Autodesk Fusion 360 part; units mm, degrees
(part 5 of 6)
  spline S189 degree 5 poles (-34.4509, 30.6181) (-34.451, 30.6199) (-34.4519, 30.6304) (-34.4535, 30.6496) (-34.4558, 30.6774) (-34.4591, 30.7139) (-34.4633, 30.7573) (-34.4677, 30.8007) (-34.4723, 30.8442) (-34.4771, 30.8876) (-34.4821, 30.9311) (-34.4873, 30.9746) (-34.4928, 31.0181) (-34.4985, 31.0616) (-34.5043, 31.1051) (-34.5104, 31.1486) (-34.5167, 31.1922) (-34.5231, 31.2358) (-34.5298, 31.2793) (-34.5367, 31.3229) (-34.5437, 31.3665) (-34.551, 31.4102) (-34.5584, 31.4538) (-34.566, 31.4974) (-34.5738, 31.541) (-34.5818, 31.5847) (-34.59, 31.6283) (-34.5984, 31.672) (-34.6069, 31.7157) (-34.6156, 31.7594) (-34.6245, 31.803) (-34.6336, 31.8467) (-34.6428, 31.8904) (-34.6522, 31.9341) (-34.6618, 31.9778) (-34.6715, 32.0215) (-34.6815, 32.0652) (-34.6916, 32.1089) (-34.7018, 32.1527) (-34.7122, 32.1964) (-34.7228, 32.2401) (-34.7336, 32.2838) (-34.7445, 32.3275) (-34.7556, 32.3713) (-34.7668, 32.415) (-34.7782, 32.4587) (-34.7897, 32.5024) (-34.7991, 32.5374) (-34.8062, 32.5636) (-34.811, 32.5811) (-34.8134, 32.5899) knots 0.354152 0.354152 0.354152 0.354152 0.354152 0.354152 0.357143 0.371429 0.385714 0.4 0.414286 0.428571 0.442857 0.457143 0.471429 0.485714 0.5 0.514286 0.528571 0.542857 0.557143 0.571429 0.585714 0.6 0.614286 0.628571 0.642857 0.657143 0.671429 0.685714 0.7 0.714286 0.728571 0.742857 0.757143 0.771429 0.785714 0.8 0.814286 0.828571 0.842857 0.857143 0.871429 0.885714 0.9 0.914286 0.928571 0.942857 0.957143 0.971429 0.985714 1 1 1 1 1 1
  arc A95 (-34.8134, 32.5899) -> (-35.5172, 32.6941) centre (-40, 0) ccw
  spline S190 degree 5 poles (-35.5172, 32.6941) (-35.5221, 32.6864) (-35.5317, 32.6711) (-35.5461, 32.648) (-35.5652, 32.6173) (-35.5889, 32.5788) (-35.6125, 32.5402) (-35.6359, 32.5016) (-35.6592, 32.463) (-35.6823, 32.4243) (-35.7053, 32.3856) (-35.7281, 32.3468) (-35.7507, 32.308) (-35.7732, 32.2692) (-35.7955, 32.2302) (-35.8177, 32.1913) (-35.8397, 32.1523) (-35.8615, 32.1132) (-35.8832, 32.0741) (-35.9047, 32.035) (-35.9261, 31.9958) (-35.9472, 31.9566) (-35.9682, 31.9173) (-35.9891, 31.878) (-36.0097, 31.8386) (-36.0302, 31.7992) (-36.0505, 31.7598) (-36.0706, 31.7203) (-36.0906, 31.6807) (-36.1103, 31.6411) (-36.1299, 31.6015) (-36.1493, 31.5618) (-36.1685, 31.5221) (-36.1875, 31.4823) (-36.2063, 31.4425) (-36.225, 31.4026) (-36.2434, 31.3627) (-36.2616, 31.3227) (-36.2797, 31.2827) (-36.2975, 31.2427) (-36.3151, 31.2026) (-36.3325, 31.1624) (-36.3497, 31.1222) (-36.3667, 31.082) (-36.3835, 31.0417) (-36.4, 31.0014) (-36.4138, 30.9674) (-36.4241, 30.9414) (-36.4312, 30.9236) (-36.435, 30.9138) (-36.4357, 30.9121) knots -1 -1 -1 -1 -1 -1 -0.985714 -0.971429 -0.957143 -0.942857 -0.928571 -0.914286 -0.9 -0.885714 -0.871429 -0.857143 -0.842857 -0.828571 -0.814286 -0.8 -0.785714 -0.771429 -0.757143 -0.742857 -0.728571 -0.714286 -0.7 -0.685714 -0.671429 -0.657143 -0.642857 -0.628571 -0.614286 -0.6 -0.585714 -0.571429 -0.557143 -0.542857 -0.528571 -0.514286 -0.5 -0.485714 -0.471429 -0.457143 -0.442857 -0.428571 -0.414286 -0.4 -0.385714 -0.371429 -0.357143 -0.354152 -0.354152 -0.354152 -0.354152 -0.354152 -0.354152
  spline S191 degree 3 poles (-36.9506, 30.5976) (-36.8858, 30.5912) (-36.8204, 30.5974) (-36.6956, 30.6347) (-36.6374, 30.6653) (-36.5533, 30.7333) (-36.5234, 30.7646) (-36.4724, 30.8341) (-36.4515, 30.872) (-36.4357, 30.9121) knots 0 0 0 0 0.019532 0.019532 0.039064 0.039064 0.051994 0.051994 0.064924 0.064924 0.064924 0.064924
  arc A96 (-36.9506, 30.5976) -> (-37.0349, 30.6059) centre (-40, 0) ccw
  spline S192 degree 3 poles (-37.4787, 31.0146) (-37.4671, 30.9505) (-37.4431, 30.8893) (-37.373, 30.7796) (-37.3276, 30.7321) (-37.2391, 30.6698) (-37.2008, 30.6497) (-37.12, 30.6197) (-37.0778, 30.6101) (-37.0349, 30.6059) knots 0 0 0 0 0.019532 0.019532 0.039064 0.039064 0.051994 0.051994 0.064924 0.064924 0.064924 0.064924
  spline S193 degree 5 poles (-37.4787, 31.0146) (-37.479, 31.0164) (-37.4809, 31.0267) (-37.4843, 31.0456) (-37.4895, 31.0731) (-37.4963, 31.1091) (-37.5047, 31.1519) (-37.5133, 31.1947) (-37.5221, 31.2374) (-37.5312, 31.2802) (-37.5404, 31.323) (-37.5499, 31.3657) (-37.5596, 31.4085) (-37.5695, 31.4512) (-37.5796, 31.494) (-37.5899, 31.5367) (-37.6004, 31.5795) (-37.6111, 31.6222) (-37.6221, 31.6649) (-37.6332, 31.7076) (-37.6445, 31.7503) (-37.6559, 31.793) (-37.6676, 31.8357) (-37.6795, 31.8784) (-37.6915, 31.921) (-37.7038, 31.9637) (-37.7162, 32.0063) (-37.7288, 32.049) (-37.7415, 32.0916) (-37.7545, 32.1342) (-37.7676, 32.1768) (-37.7809, 32.2194) (-37.7944, 32.262) (-37.808, 32.3045) (-37.8219, 32.3471) (-37.8359, 32.3896) (-37.85, 32.4321) (-37.8643, 32.4746) (-37.8788, 32.5171) (-37.8935, 32.5596) (-37.9083, 32.6021) (-37.9233, 32.6446) (-37.9384, 32.687) (-37.9537, 32.7294) (-37.9692, 32.7718) (-37.9848, 32.8142) (-38.0006, 32.8566) (-38.0134, 32.8905) (-38.023, 32.9159) (-38.0295, 32.9328) (-38.0327, 32.9413) knots 0.354152 0.354152 0.354152 0.354152 0.354152 0.354152 0.357143 0.371429 0.385714 0.4 0.414286 0.428571 0.442857 0.457143 0.471429 0.485714 0.5 0.514286 0.528571 0.542857 0.557143 0.571429 0.585714 0.6 0.614286 0.628571 0.642857 0.657143 0.671429 0.685714 0.7 0.714286 0.728571 0.742857 0.757143 0.771429 0.785714 0.8 0.814286 0.828571 0.842857 0.857143 0.871429 0.885714 0.9 0.914286 0.928571 0.942857 0.957143 0.971429 0.985714 1 1 1 1 1 1
  arc A97 (-38.0327, 32.9413) -> (-38.7434, 32.9761) centre (-40, 0) ccw
  spline S194 degree 5 poles (-38.7434, 32.9761) (-38.7475, 32.968) (-38.7555, 32.9517) (-38.7676, 32.9274) (-38.7836, 32.8949) (-38.8034, 32.8543) (-38.8231, 32.8136) (-38.8427, 32.7729) (-38.862, 32.7322) (-38.8812, 32.6914) (-38.9003, 32.6506) (-38.9192, 32.6098) (-38.9379, 32.5689) (-38.9565, 32.5281) (-38.9749, 32.4872) (-38.9931, 32.4462) (-39.0112, 32.4052) (-39.0291, 32.3642) (-39.0469, 32.3232) (-39.0644, 32.2822) (-39.0818, 32.2411) (-39.099, 32.2) (-39.1161, 32.1588) (-39.133, 32.1176) (-39.1497, 32.0764) (-39.1662, 32.0352) (-39.1825, 31.9939) (-39.1987, 31.9527) (-39.2146, 31.9113) (-39.2304, 31.87) (-39.246, 31.8286) (-39.2614, 31.7872) (-39.2766, 31.7458) (-39.2917, 31.7044) (-39.3065, 31.6629) (-39.3211, 31.6214) (-39.3356, 31.5799) (-39.3498, 31.5383) (-39.3638, 31.4967) (-39.3776, 31.4551) (-39.3912, 31.4135) (-39.4046, 31.3718) (-39.4178, 31.3302) (-39.4308, 31.2885) (-39.4435, 31.2467) (-39.456, 31.205) (-39.4664, 31.1698) (-39.4741, 31.143) (-39.4794, 31.1245) (-39.4823, 31.1144) (-39.4828, 31.1126) knots -1 -1 -1 -1 -1 -1 -0.985714 -0.971429 -0.957143 -0.942857 -0.928571 -0.914286 -0.9 -0.885714 -0.871429 -0.857143 -0.842857 -0.828571 -0.814286 -0.8 -0.785714 -0.771429 -0.757143 -0.742857 -0.728571 -0.714286 -0.7 -0.685714 -0.671429 -0.657143 -0.642857 -0.628571 -0.614286 -0.6 -0.585714 -0.571429 -0.557143 -0.542857 -0.528571 -0.514286 -0.5 -0.485714 -0.471429 -0.457143 -0.442857 -0.428571 -0.414286 -0.4 -0.385714 -0.371429 -0.357143 -0.354152 -0.354152 -0.354152 -0.354152 -0.354152 -0.354152
  spline S195 degree 3 poles (-39.9643, 30.7492) (-39.8992, 30.7491) (-39.8347, 30.7617) (-39.7142, 30.811) (-39.6593, 30.8472) (-39.5822, 30.9231) (-39.5556, 30.9572) (-39.5116, 31.0314) (-39.4946, 31.0712) (-39.4828, 31.1126) knots 0 0 0 0 0.019532 0.019532 0.039064 0.039064 0.051994 0.051994 0.064924 0.064924 0.064924 0.064924
  arc A98 (-39.9643, 30.7492) -> (-40.0491, 30.7492) centre (-40, 0) ccw
  spline S196 degree 3 poles (-40.5308, 31.1124) (-40.513, 31.0498) (-40.4831, 30.9912) (-40.4026, 30.8889) (-40.3527, 30.846) (-40.2586, 30.7928) (-40.2185, 30.7765) (-40.1351, 30.7546) (-40.0922, 30.7491) (-40.0491, 30.7492) knots 0 0 0 0 0.019532 0.019532 0.039064 0.039064 0.051994 0.051994 0.064924 0.064924 0.064924 0.064924
  spline S197 degree 5 poles (-40.5308, 31.1124) (-40.5313, 31.1141) (-40.5342, 31.1242) (-40.5395, 31.1427) (-40.5472, 31.1696) (-40.5576, 31.2047) (-40.5701, 31.2465) (-40.5829, 31.2882) (-40.5959, 31.3299) (-40.6091, 31.3716) (-40.6225, 31.4132) (-40.6361, 31.4549) (-40.6499, 31.4965) (-40.664, 31.538) (-40.6782, 31.5796) (-40.6927, 31.6211) (-40.7073, 31.6626) (-40.7222, 31.7041) (-40.7372, 31.7455) (-40.7524, 31.7869) (-40.7679, 31.8283) (-40.7835, 31.8697) (-40.7993, 31.911) (-40.8153, 31.9523) (-40.8314, 31.9936) (-40.8478, 32.0348) (-40.8643, 32.0761) (-40.8811, 32.1173) (-40.8979, 32.1584) (-40.915, 32.1996) (-40.9322, 32.2407) (-40.9497, 32.2817) (-40.9672, 32.3228) (-40.985, 32.3638) (-41.0029, 32.4048) (-41.021, 32.4458) (-41.0393, 32.4867) (-41.0577, 32.5276) (-41.0763, 32.5685) (-41.095, 32.6093) (-41.1139, 32.6501) (-41.133, 32.6909) (-41.1522, 32.7317) (-41.1716, 32.7724) (-41.1912, 32.8131) (-41.2109, 32.8537) (-41.2308, 32.8944) (-41.2468, 32.9268) (-41.2588, 32.9512) (-41.2669, 32.9674) (-41.271, 32.9755) knots 0.354152 0.354152 0.354152 0.354152 0.354152 0.354152 0.357143 0.371429 0.385714 0.4 0.414286 0.428571 0.442857 0.457143 0.471429 0.485714 0.5 0.514286 0.528571 0.542857 0.557143 0.571429 0.585714 0.6 0.614286 0.628571 0.642857 0.657143 0.671429 0.685714 0.7 0.714286 0.728571 0.742857 0.757143 0.771429 0.785714 0.8 0.814286 0.828571 0.842857 0.857143 0.871429 0.885714 0.9 0.914286 0.928571 0.942857 0.957143 0.971429 0.985714 1 1 1 1 1 1
  arc A99 (-41.271, 32.9755) -> (-41.9817, 32.9404) centre (-40, 0) ccw
  spline S198 degree 5 poles (-41.9817, 32.9404) (-41.9849, 32.932) (-41.9914, 32.915) (-42.001, 32.8896) (-42.0137, 32.8557) (-42.0295, 32.8133) (-42.0451, 32.7709) (-42.0605, 32.7285) (-42.0758, 32.6861) (-42.091, 32.6436) (-42.1059, 32.6012) (-42.1207, 32.5587) (-42.1354, 32.5162) (-42.1498, 32.4737) (-42.1641, 32.4312) (-42.1783, 32.3887) (-42.1922, 32.3461) (-42.206, 32.3036) (-42.2197, 32.261) (-42.2331, 32.2184) (-42.2464, 32.1758) (-42.2595, 32.1332) (-42.2725, 32.0906) (-42.2852, 32.048) (-42.2978, 32.0053) (-42.3102, 31.9627) (-42.3224, 31.92) (-42.3344, 31.8773) (-42.3463, 31.8347) (-42.3579, 31.792) (-42.3694, 31.7493) (-42.3807, 31.7066) (-42.3918, 31.6639) (-42.4027, 31.6211) (-42.4133, 31.5784) (-42.4238, 31.5357) (-42.4341, 31.4929) (-42.4442, 31.4502) (-42.4541, 31.4074) (-42.4638, 31.3647) (-42.4732, 31.3219) (-42.4825, 31.2791) (-42.4915, 31.2364) (-42.5003, 31.1936) (-42.5089, 31.1508) (-42.5173, 31.108) (-42.5241, 31.072) (-42.5292, 31.0445) (-42.5326, 31.0256) (-42.5345, 31.0153) (-42.5348, 31.0135) knots -1 -1 -1 -1 -1 -1 -0.985714 -0.971429 -0.957143 -0.942857 -0.928571 -0.914286 -0.9 -0.885714 -0.871429 -0.857143 -0.842857 -0.828571 -0.814286 -0.8 -0.785714 -0.771429 -0.757143 -0.742857 -0.728571 -0.714286 -0.7 -0.685714 -0.671429 -0.657143 -0.642857 -0.628571 -0.614286 -0.6 -0.585714 -0.571429 -0.557143 -0.542857 -0.528571 -0.514286 -0.5 -0.485714 -0.471429 -0.457143 -0.442857 -0.428571 -0.414286 -0.4 -0.385714 -0.371429 -0.357143 -0.354152 -0.354152 -0.354152 -0.354152 -0.354152 -0.354152
  spline S199 degree 3 poles (-42.9785, 30.6046) (-42.9137, 30.6109) (-42.8507, 30.6298) (-42.7356, 30.6907) (-42.6845, 30.7321) (-42.6153, 30.8152) (-42.5921, 30.8517) (-42.5556, 30.9298) (-42.5425, 30.9711) (-42.5348, 31.0135) knots 0 0 0 0 0.019532 0.019532 0.039064 0.039064 0.051994 0.051994 0.064924 0.064924 0.064924 0.064924
  arc A100 (-42.9785, 30.6046) -> (-43.0628, 30.5963) centre (-40, 0) ccw
  spline S200 degree 3 poles (-43.5778, 30.9105) (-43.5539, 30.85) (-43.5185, 30.7946) (-43.4283, 30.7007) (-43.3745, 30.6629) (-43.2755, 30.6191) (-43.234, 30.6069) (-43.1489, 30.5933) (-43.1057, 30.592) (-43.0628, 30.5963) knots 0 0 0 0 0.019532 0.019532 0.039064 0.039064 0.051994 0.051994 0.064924 0.064924 0.064924 0.064924
  spline S201 degree 5 poles (-43.5778, 30.9105) (-43.5785, 30.9122) (-43.5823, 30.922) (-43.5894, 30.9399) (-43.5998, 30.9658) (-43.6135, 30.9998) (-43.6301, 31.0401) (-43.6469, 31.0804) (-43.6639, 31.1206) (-43.6811, 31.1608) (-43.6985, 31.201) (-43.7161, 31.241) (-43.734, 31.2811) (-43.752, 31.3211) (-43.7703, 31.361) (-43.7887, 31.4009) (-43.8074, 31.4408) (-43.8262, 31.4806) (-43.8453, 31.5204) (-43.8645, 31.5601) (-43.8839, 31.5998) (-43.9035, 31.6394) (-43.9233, 31.679) (-43.9432, 31.7185) (-43.9634, 31.758) (-43.9837, 31.7975) (-44.0042, 31.8369) (-44.0248, 31.8762) (-44.0457, 31.9156) (-44.0667, 31.9548) (-44.0879, 31.994) (-44.1093, 32.0332) (-44.1308, 32.0723) (-44.1525, 32.1114) (-44.1743, 32.1505) (-44.1963, 32.1895) (-44.2185, 32.2284) (-44.2409, 32.2673) (-44.2634, 32.3062) (-44.286, 32.345) (-44.3089, 32.3837) (-44.3318, 32.4224) (-44.355, 32.4611) (-44.3783, 32.4997) (-44.4017, 32.5383) (-44.4253, 32.5768) (-44.449, 32.6153) (-44.4682, 32.6461) (-44.4826, 32.6691) (-44.4922, 32.6845) (-44.497, 32.6922) knots 0.354152 0.354152 0.354152 0.354152 0.354152 0.354152 0.357143 0.371429 0.385714 0.4 0.414286 0.428571 0.442857 0.457143 0.471429 0.485714 0.5 0.514286 0.528571 0.542857 0.557143 0.571429 0.585714 0.6 0.614286 0.628571 0.642857 0.657143 0.671429 0.685714 0.7 0.714286 0.728571 0.742857 0.757143 0.771429 0.785714 0.8 0.814286 0.828571 0.842857 0.857143 0.871429 0.885714 0.9 0.914286 0.928571 0.942857 0.957143 0.971429 0.985714 1 1 1 1 1 1
  arc A101 (-44.497, 32.6922) -> (-45.2009, 32.5876) centre (-40, 0) ccw
  spline S202 degree 5 poles (-45.2009, 32.5876) (-45.2033, 32.5788) (-45.208, 32.5614) (-45.2151, 32.5351) (-45.2245, 32.5001) (-45.236, 32.4564) (-45.2474, 32.4127) (-45.2586, 32.369) (-45.2696, 32.3252) (-45.2805, 32.2815) (-45.2913, 32.2378) (-45.3018, 32.1941) (-45.3122, 32.1503) (-45.3225, 32.1066) (-45.3325, 32.0629) (-45.3424, 32.0192) (-45.3522, 31.9755) (-45.3617, 31.9318) (-45.3711, 31.8881) (-45.3803, 31.8444) (-45.3894, 31.8007) (-45.3983, 31.757) (-45.4069, 31.7133) (-45.4155, 31.6697) (-45.4238, 31.626) (-45.432, 31.5823) (-45.4399, 31.5387) (-45.4477, 31.495) (-45.4553, 31.4514) (-45.4627, 31.4078) (-45.47, 31.3642) (-45.477, 31.3206) (-45.4838, 31.277) (-45.4905, 31.2334) (-45.4969, 31.1898) (-45.5032, 31.1462) (-45.5093, 31.1027) (-45.5151, 31.0592) (-45.5207, 31.0156) (-45.5262, 30.9721) (-45.5314, 30.9287) (-45.5364, 30.8852) (-45.5412, 30.8417) (-45.5458, 30.7983) (-45.5501, 30.7549) (-45.5543, 30.7115) (-45.5575, 30.675) (-45.5599, 30.6471) (-45.5615, 30.628) (-45.5623, 30.6175) (-45.5625, 30.6157) knots -1 -1 -1 -1 -1 -1 -0.985714 -0.971429 -0.957143 -0.942857 -0.928571 -0.914286 -0.9 -0.885714 -0.871429 -0.857143 -0.842857 -0.828571 -0.814286 -0.8 -0.785714 -0.771429 -0.757143 -0.742857 -0.728571 -0.714286 -0.7 -0.685714 -0.671429 -0.657143 -0.642857 -0.628571 -0.614286 -0.6 -0.585714 -0.571429 -0.557143 -0.542857 -0.528571 -0.514286 -0.5 -0.485714 -0.471429 -0.457143 -0.442857 -0.428571 -0.414286 -0.4 -0.385714 -0.371429 -0.357143 -0.354152 -0.354152 -0.354152 -0.354152 -0.354152 -0.354152
  spline S203 degree 3 poles (-45.9639, 30.1653) (-45.9, 30.1779) (-45.8392, 30.2029) (-45.7306, 30.2748) (-45.6839, 30.321) (-45.6231, 30.4105) (-45.6036, 30.4491) (-45.5749, 30.5304) (-45.5659, 30.5727) (-45.5625, 30.6157) knots 0 0 0 0 0.019532 0.019532 0.039064 0.039064 0.051994 0.051994 0.064924 0.064924 0.064924 0.064924
  arc A102 (-45.9639, 30.1653) -> (-46.047, 30.1488) centre (-40, 0) ccw
  spline S204 degree 3 poles (-46.5903, 30.411) (-46.5606, 30.3531) (-46.5199, 30.3015) (-46.421, 30.2168) (-46.3637, 30.1845) (-46.261, 30.1506) (-46.2185, 30.1425) (-46.1324, 30.1373) (-46.0892, 30.1403) (-46.047, 30.1488) knots 0 0 0 0 0.019532 0.019532 0.039064 0.039064 0.051994 0.051994 0.064924 0.064924 0.064924 0.064924
  spline S205 degree 5 poles (-46.5903, 30.411) (-46.5912, 30.4126) (-46.5959, 30.422) (-46.6047, 30.4391) (-46.6176, 30.4639) (-46.6346, 30.4964) (-46.6551, 30.5349) (-46.6757, 30.5733) (-46.6966, 30.6117) (-46.7176, 30.65) (-46.7389, 30.6882) (-46.7604, 30.7264) (-46.7821, 30.7645) (-46.804, 30.8025) (-46.8261, 30.8405) (-46.8483, 30.8784) (-46.8708, 30.9162) (-46.8934, 30.954) (-46.9163, 30.9917) (-46.9393, 31.0293) (-46.9625, 31.0669) (-46.9859, 31.1045) (-47.0095, 31.1419) (-47.0332, 31.1793) (-47.0571, 31.2166) (-47.0812, 31.2539) (-47.1055, 31.2911) (-47.1299, 31.3282) (-47.1545, 31.3653) (-47.1792, 31.4023) (-47.2042, 31.4393) (-47.2293, 31.4762) (-47.2545, 31.513) (-47.2799, 31.5498) (-47.3055, 31.5865) (-47.3313, 31.6231) (-47.3571, 31.6597) (-47.3832, 31.6963) (-47.4094, 31.7327) (-47.4358, 31.7691) (-47.4623, 31.8055) (-47.4889, 31.8417) (-47.5157, 31.8779) (-47.5427, 31.9141) (-47.5698, 31.9502) (-47.5971, 31.9862) (-47.6245, 32.0222) (-47.6465, 32.0509) (-47.6631, 32.0724) (-47.6742, 32.0868) (-47.6798, 32.0939) knots 0.354152 0.354152 0.354152 0.354152 0.354152 0.354152 0.357143 0.371429 0.385714 0.4 0.414286 0.428571 0.442857 0.457143 0.471429 0.485714 0.5 0.514286 0.528571 0.542857 0.557143 0.571429 0.585714 0.6 0.614286 0.628571 0.642857 0.657143 0.671429 0.685714 0.7 0.714286 0.728571 0.742857 0.757143 0.771429 0.785714 0.8 0.814286 0.828571 0.842857 0.857143 0.871429 0.885714 0.9 0.914286 0.928571 0.942857 0.957143 0.971429 0.985714 1 1 1 1 1 1
  arc A103 (-47.6798, 32.0939) -> (-48.37, 31.9209) centre (-40, 0) ccw
  spline S206 degree 5 poles (-48.37, 31.9209) (-48.3715, 31.912) (-48.3745, 31.8941) (-48.379, 31.8673) (-48.3849, 31.8316) (-48.3921, 31.7869) (-48.3991, 31.7423) (-48.406, 31.6977) (-48.4127, 31.6531) (-48.4192, 31.6085) (-48.4256, 31.5639) (-48.4319, 31.5194) (-48.4379, 31.4748) (-48.4438, 31.4303) (-48.4496, 31.3858) (-48.4551, 31.3414) (-48.4605, 31.2969) (-48.4658, 31.2525) (-48.4708, 31.2081) (-48.4757, 31.1637) (-48.4804, 31.1193) (-48.485, 31.075) (-48.4894, 31.0306) (-48.4936, 30.9863) (-48.4976, 30.9421) (-48.5014, 30.8978) (-48.5051, 30.8536) (-48.5085, 30.8094) (-48.5118, 30.7652) (-48.5149, 30.7211) (-48.5178, 30.677) (-48.5206, 30.6329) (-48.5231, 30.5888) (-48.5255, 30.5448) (-48.5276, 30.5008) (-48.5296, 30.4569) (-48.5313, 30.4129) (-48.5329, 30.369) (-48.5342, 30.3252) (-48.5354, 30.2813) (-48.5363, 30.2376) (-48.537, 30.1938) (-48.5375, 30.1501) (-48.5378, 30.1064) (-48.5379, 30.0628) (-48.5378, 30.0192) (-48.5375, 29.9825) (-48.5371, 29.9546) (-48.5368, 29.9354) (-48.5366, 29.9249) (-48.5366, 29.9231) knots -1 -1 -1 -1 -1 -1 -0.985714 -0.971429 -0.957143 -0.942857 -0.928571 -0.914286 -0.9 -0.885714 -0.871429 -0.857143 -0.842857 -0.828571 -0.814286 -0.8 -0.785714 -0.771429 -0.757143 -0.742857 -0.728571 -0.714286 -0.7 -0.685714 -0.671429 -0.657143 -0.642857 -0.628571 -0.614286 -0.6 -0.585714 -0.571429 -0.557143 -0.542857 -0.528571 -0.514286 -0.5 -0.485714 -0.471429 -0.457143 -0.442857 -0.428571 -0.414286 -0.4 -0.385714 -0.371429 -0.357143 -0.354152 -0.354152 -0.354152 -0.354152 -0.354152 -0.354152
  spline S207 degree 3 poles (-48.8919, 29.4355) (-48.8296, 29.4543) (-48.7715, 29.4851) (-48.6705, 29.5673) (-48.6285, 29.6178) (-48.5767, 29.7129) (-48.5611, 29.7532) (-48.5406, 29.837) (-48.5358, 29.88) (-48.5366, 29.9231) knots 0 0 0 0 0.019532 0.019532 0.039064 0.039064 0.051994 0.051994 0.064924 0.064924 0.064924 0.064924
  arc A104 (-48.8919, 29.4355) -> (-48.973, 29.4109) centre (-40, 0) ccw
  spline S208 degree 3 poles (-49.5394, 29.6186) (-49.5042, 29.5639) (-49.4586, 29.5165) (-49.3518, 29.4419) (-49.2917, 29.4154) (-49.1861, 29.3918) (-49.143, 29.3878) (-49.0569, 29.3911) (-49.0142, 29.3983) (-48.973, 29.4109) knots 0 0 0 0 0.019532 0.019532 0.039064 0.039064 0.051994 0.051994 0.064924 0.064924 0.064924 0.064924
  spline S209 degree 5 poles (-49.5394, 29.6186) (-49.5404, 29.6201) (-49.5461, 29.629) (-49.5565, 29.6451) (-49.5717, 29.6685) (-49.5918, 29.6992) (-49.6159, 29.7355) (-49.6403, 29.7717) (-49.6648, 29.8079) (-49.6895, 29.8439) (-49.7144, 29.8799) (-49.7396, 29.9158) (-49.7649, 29.9516) (-49.7904, 29.9873) (-49.8161, 30.0229) (-49.842, 30.0584) (-49.868, 30.0939) (-49.8943, 30.1293) (-49.9207, 30.1646) (-49.9473, 30.1998) (-49.9741, 30.2349) (-50.001, 30.2699) (-50.0281, 30.3049) (-50.0554, 30.3398) (-50.0829, 30.3746) (-50.1105, 30.4093) (-50.1383, 30.444) (-50.1663, 30.4785) (-50.1944, 30.513) (-50.2226, 30.5474) (-50.2511, 30.5818) (-50.2797, 30.616) (-50.3084, 30.6502) (-50.3373, 30.6843) (-50.3664, 30.7183) (-50.3956, 30.7523) (-50.4249, 30.7862) (-50.4544, 30.8199) (-50.4841, 30.8537) (-50.5139, 30.8873) (-50.5438, 30.9209) (-50.5739, 30.9544) (-50.6041, 30.9878) (-50.6345, 31.0211) (-50.665, 31.0544) (-50.6957, 31.0876) (-50.7265, 31.1207) (-50.7512, 31.1471) (-50.7699, 31.1669) (-50.7823, 31.1801) (-50.7885, 31.1867) knots 0.354152 0.354152 0.354152 0.354152 0.354152 0.354152 0.357143 0.371429 0.385714 0.4 0.414286 0.428571 0.442857 0.457143 0.471429 0.485714 0.5 0.514286 0.528571 0.542857 0.557143 0.571429 0.585714 0.6 0.614286 0.628571 0.642857 0.657143 0.671429 0.685714 0.7 0.714286 0.728571 0.742857 0.757143 0.771429 0.785714 0.8 0.814286 0.828571 0.842857 0.857143 0.871429 0.885714 0.9 0.914286 0.928571 0.942857 0.957143 0.971429 0.985714 1 1 1 1 1 1
  arc A105 (-50.7885, 31.1867) -> (-51.4585, 30.9468) centre (-40, 0) ccw
  spline S210 degree 5 poles (-51.4585, 30.9468) (-51.4591, 30.9377) (-51.4603, 30.9197) (-51.4622, 30.8926) (-51.4645, 30.8564) (-51.4673, 30.8113) (-51.4699, 30.7662) (-51.4724, 30.7211) (-51.4747, 30.6761) (-51.4769, 30.6311) (-51.4789, 30.5861) (-51.4807, 30.5411) (-51.4824, 30.4962) (-51.4839, 30.4513) (-51.4852, 30.4065) (-51.4864, 30.3617) (-51.4874, 30.3169) (-51.4883, 30.2722) (-51.489, 30.2275) (-51.4895, 30.1829) (-51.4898, 30.1382) (-51.49, 30.0937) (-51.49, 30.0491) (-51.4898, 30.0046) (-51.4895, 29.9602) (-51.489, 29.9158) (-51.4883, 29.8714) (-51.4874, 29.8271) (-51.4864, 29.7828) (-51.4851, 29.7386) (-51.4837, 29.6944) (-51.4821, 29.6502) (-51.4803, 29.6061) (-51.4783, 29.5621) (-51.4762, 29.5181) (-51.4738, 29.4742) (-51.4712, 29.4303) (-51.4685, 29.3864) (-51.4655, 29.3426) (-51.4624, 29.2989) (-51.459, 29.2553) (-51.4554, 29.2116) (-51.4517, 29.1681) (-51.4477, 29.1246) (-51.4435, 29.0812) (-51.4391, 29.0378) (-51.4351, 29.0013) (-51.432, 28.9736) (-51.4299, 28.9545) (-51.4286, 28.944) (-51.4284, 28.9422) knots -1 -1 -1 -1 -1 -1 -0.985714 -0.971429 -0.957143 -0.942857 -0.928571 -0.914286 -0.9 -0.885714 -0.871429 -0.857143 -0.842857 -0.828571 -0.814286 -0.8 -0.785714 -0.771429 -0.757143 -0.742857 -0.728571 -0.714286 -0.7 -0.685714 -0.671429 -0.657143 -0.642857 -0.628571 -0.614286 -0.6 -0.585714 -0.571429 -0.557143 -0.542857 -0.528571 -0.514286 -0.5 -0.485714 -0.471429 -0.457143 -0.442857 -0.428571 -0.414286 -0.4 -0.385714 -0.371429 -0.357143 -0.354152 -0.354152 -0.354152 -0.354152 -0.354152 -0.354152
  spline S211 degree 3 poles (-51.7343, 28.4222) (-51.6741, 28.447) (-51.6193, 28.4834) (-51.5268, 28.5751) (-51.49, 28.6295) (-51.4478, 28.7291) (-51.4362, 28.7708) (-51.424, 28.8562) (-51.4234, 28.8994) (-51.4284, 28.9422) knots 0 0 0 0 0.019532 0.019532 0.039064 0.039064 0.051994 0.051994 0.064924 0.064924 0.064924 0.064924
  arc A106 (-51.7343, 28.4222) -> (-51.8125, 28.3897) centre (-40, 0) ccw
  spline S212 degree 3 poles (-52.3966, 28.541) (-52.3562, 28.4899) (-52.3062, 28.4473) (-52.1926, 28.3835) (-52.1302, 28.363) (-52.0228, 28.3499) (-51.9795, 28.3502) (-51.8941, 28.3618) (-51.8523, 28.3732) (-51.8125, 28.3897) knots 0 0 0 0 0.019532 0.019532 0.039064 0.039064 0.051994 0.051994 0.064924 0.064924 0.064924 0.064924
  spline S213 degree 5 poles (-52.3966, 28.541) (-52.3977, 28.5424) (-52.4042, 28.5506) (-52.4162, 28.5657) (-52.4337, 28.5875) (-52.4567, 28.616) (-52.4842, 28.6498) (-52.512, 28.6835) (-52.5399, 28.717) (-52.5681, 28.7505) (-52.5964, 28.7838) (-52.6249, 28.8171) (-52.6536, 28.8502) (-52.6825, 28.8832) (-52.7116, 28.9162) (-52.7408, 28.949) (-52.7702, 28.9817) (-52.7998, 29.0144) (-52.8296, 29.0469) (-52.8595, 29.0793) (-52.8896, 29.1117) (-52.9198, 29.1439) (-52.9503, 29.176) (-52.9808, 29.2081) (-53.0116, 29.24) (-53.0425, 29.2719) (-53.0735, 29.3036) (-53.1047, 29.3353) (-53.1361, 29.3669) (-53.1676, 29.3984) (-53.1993, 29.4297) (-53.2311, 29.461) (-53.263, 29.4922) (-53.2951, 29.5233) (-53.3274, 29.5543) (-53.3598, 29.5853) (-53.3923, 29.6161) (-53.425, 29.6468) (-53.4578, 29.6775) (-53.4907, 29.708) (-53.5238, 29.7385) (-53.557, 29.7689) (-53.5904, 29.7992) (-53.6239, 29.8294) (-53.6575, 29.8595) (-53.6913, 29.8895) (-53.7252, 29.9194) (-53.7524, 29.9433) (-53.7729, 29.9612) (-53.7866, 29.9731) (-53.7934, 29.979) knots 0.354152 0.354152 0.354152 0.354152 0.354152 0.354152 0.357143 0.371429 0.385714 0.4 0.414286 0.428571 0.442857 0.457143 0.471429 0.485714 0.5 0.514286 0.528571 0.542857 0.557143 0.571429 0.585714 0.6 0.614286 0.628571 0.642857 0.657143 0.671429 0.685714 0.7 0.714286 0.728571 0.742857 0.757143 0.771429 0.785714 0.8 0.814286 0.828571 0.842857 0.857143 0.871429 0.885714 0.9 0.914286 0.928571 0.942857 0.957143 0.971429 0.985714 1 1 1 1 1 1
  arc A107 (-53.7934, 29.979) -> (-54.4366, 29.6746) centre (-40, 0) ccw
  spline S214 degree 5 poles (-54.4366, 29.6746) (-54.4363, 29.6656) (-54.4358, 29.6475) (-54.435, 29.6203) (-54.4338, 29.5841) (-54.4321, 29.5389) (-54.4303, 29.4938) (-54.4284, 29.4487) (-54.4262, 29.4036) (-54.424, 29.3586) (-54.4215, 29.3137) (-54.419, 29.2688) (-54.4162, 29.2239) (-54.4133, 29.1791) (-54.4103, 29.1343) (-54.4071, 29.0896) (-54.4037, 29.045) (-54.4002, 29.0004) (-54.3965, 28.9558) (-54.3926, 28.9113) (-54.3886, 28.8669) (-54.3844, 28.8225) (-54.38, 28.7782) (-54.3755, 28.7339) (-54.3708, 28.6897) (-54.3659, 28.6456) (-54.3609, 28.6015) (-54.3557, 28.5575) (-54.3503, 28.5135) (-54.3447, 28.4696) (-54.339, 28.4258) (-54.333, 28.382) (-54.3269, 28.3383) (-54.3206, 28.2947) (-54.3142, 28.2511) (-54.3075, 28.2076) (-54.3007, 28.1642) (-54.2936, 28.1208) (-54.2864, 28.0775) (-54.279, 28.0343) (-54.2713, 27.9912) (-54.2635, 27.9482) (-54.2555, 27.9052) (-54.2473, 27.8623) (-54.2388, 27.8195) (-54.2302, 27.7767) (-54.2227, 27.7409) (-54.2169, 27.7135) (-54.2129, 27.6947) (-54.2106, 27.6845) (-54.2102, 27.6827) knots -1 -1 -1 -1 -1 -1 -0.985714 -0.971429 -0.957143 -0.942857 -0.928571 -0.914286 -0.9 -0.885714 -0.871429 -0.857143 -0.842857 -0.828571 -0.814286 -0.8 -0.785714 -0.771429 -0.757143 -0.742857 -0.728571 -0.714286 -0.7 -0.685714 -0.671429 -0.657143 -0.642857 -0.628571 -0.614286 -0.6 -0.585714 -0.571429 -0.557143 -0.542857 -0.528571 -0.514286 -0.5 -0.485714 -0.471429 -0.457143 -0.442857 -0.428571 -0.414286 -0.4 -0.385714 -0.371429 -0.357143 -0.354152 -0.354152 -0.354152 -0.354152 -0.354152 -0.354152
  spline S215 degree 3 poles (-54.4636, 27.1352) (-54.4062, 27.1658) (-54.3552, 27.2073) (-54.2722, 27.3076) (-54.2409, 27.3654) (-54.2086, 27.4687) (-54.2012, 27.5113) (-54.1974, 27.5975) (-54.2011, 27.6406) (-54.2102, 27.6827) knots 0 0 0 0 0.019532 0.019532 0.039064 0.039064 0.051994 0.051994 0.064924 0.064924 0.064924 0.064924
  arc A108 (-54.4636, 27.1352) -> (-54.5383, 27.0952) centre (-40, 0) ccw
  spline S216 degree 3 poles (-55.1344, 27.1885) (-55.0892, 27.1416) (-55.0352, 27.1041) (-54.916, 27.0518) (-54.8518, 27.0375) (-54.7436, 27.0349) (-54.7006, 27.0394) (-54.6168, 27.0594) (-54.5763, 27.0748) (-54.5383, 27.0952) knots 0 0 0 0 0.019532 0.019532 0.039064 0.039064 0.051994 0.051994 0.064924 0.064924 0.064924 0.064924
  spline S217 degree 5 poles (-55.1344, 27.1885) (-55.1357, 27.1898) (-55.143, 27.1973) (-55.1563, 27.2111) (-55.1758, 27.2311) (-55.2016, 27.2573) (-55.2323, 27.2882) (-55.2632, 27.319) (-55.2943, 27.3496) (-55.3256, 27.3802) (-55.3571, 27.4106) (-55.3887, 27.4409) (-55.4205, 27.471) (-55.4525, 27.5011) (-55.4846, 27.531) (-55.517, 27.5608) (-55.5494, 27.5905) (-55.5821, 27.6201) (-55.6149, 27.6495) (-55.6478, 27.6789) (-55.681, 27.7081) (-55.7142, 27.7372) (-55.7477, 27.7662) (-55.7812, 27.7951) (-55.8149, 27.8239) (-55.8488, 27.8526) (-55.8828, 27.8811) (-55.917, 27.9096) (-55.9513, 27.9379) (-55.9857, 27.9661) (-56.0203, 27.9943) (-56.055, 28.0223) (-56.0899, 28.0502) (-56.1249, 28.078) (-56.16, 28.1057) (-56.1953, 28.1333) (-56.2307, 28.1608) (-56.2662, 28.1882) (-56.3019, 28.2155) (-56.3377, 28.2427) (-56.3736, 28.2697) (-56.4096, 28.2967) (-56.4458, 28.3236) (-56.4821, 28.3504) (-56.5185, 28.377) (-56.5551, 28.4036) (-56.5917, 28.4301) (-56.6212, 28.4512) (-56.6433, 28.4669) (-56.6581, 28.4774) (-56.6655, 28.4827) knots 0.354152 0.354152 0.354152 0.354152 0.354152 0.354152 0.357143 0.371429 0.385714 0.4 0.414286 0.428571 0.442857 0.457143 0.471429 0.485714 0.5 0.514286 0.528571 0.542857 0.557143 0.571429 0.585714 0.6 0.614286 0.628571 0.642857 0.657143 0.671429 0.685714 0.7 0.714286 0.728571 0.742857 0.757143 0.771429 0.785714 0.8 0.814286 0.828571 0.842857 0.857143 0.871429 0.885714 0.9 0.914286 0.928571 0.942857 0.957143 0.971429 0.985714 1 1 1 1 1 1
  arc A109 (-56.6655, 28.4827) -> (-57.2757, 28.1167) centre (-40, 0) ccw
  spline S218 degree 5 poles (-57.2757, 28.1167) (-57.2746, 28.1077) (-57.2723, 28.0897) (-57.2688, 28.0628) (-57.264, 28.0269) (-57.258, 27.9821) (-57.2517, 27.9373) (-57.2454, 27.8927) (-57.2388, 27.848) (-57.2322, 27.8035) (-57.2253, 27.759) (-57.2184, 27.7145) (-57.2113, 27.6701) (-57.204, 27.6258) (-57.1966, 27.5816) (-57.189, 27.5374) (-57.1812, 27.4933) (-57.1734, 27.4493) (-57.1653, 27.4053) (-57.1571, 27.3614) (-57.1487, 27.3176) (-57.1402, 27.2738) (-57.1315, 27.2301) (-57.1227, 27.1865) (-57.1137, 27.143) (-57.1045, 27.0995) (-57.0952, 27.0562) (-57.0857, 27.0129) (-57.076, 26.9696) (-57.0661, 26.9265) (-57.0561, 26.8834) (-57.0459, 26.8405) (-57.0356, 26.7976) (-57.025, 26.7548) (-57.0143, 26.712) (-57.0034, 26.6694) (-56.9924, 26.6268) (-56.9811, 26.5844) (-56.9697, 26.542) (-56.9581, 26.4998) (-56.9462, 26.4576) (-56.9342, 26.4155) (-56.922, 26.3735) (-56.9096, 26.3316) (-56.897, 26.2899) (-56.8842, 26.2482) (-56.8733, 26.2132) (-56.8648, 26.1866) (-56.859, 26.1683) (-56.8557, 26.1583) (-56.8552, 26.1565) knots -1 -1 -1 -1 -1 -1 -0.985714 -0.971429 -0.957143 -0.942857 -0.928571 -0.914286 -0.9 -0.885714 -0.871429 -0.857143 -0.842857 -0.828571 -0.814286 -0.8 -0.785714 -0.771429 -0.757143 -0.742857 -0.728571 -0.714286 -0.7 -0.685714 -0.671429 -0.657143 -0.642857 -0.628571 -0.614286 -0.6 -0.585714 -0.571429 -0.557143 -0.542857 -0.528571 -0.514286 -0.5 -0.485714 -0.471429 -0.457143 -0.442857 -0.428571 -0.414286 -0.4 -0.385714 -0.371429 -0.357143 -0.354152 -0.354152 -0.354152 -0.354152 -0.354152 -0.354152
  spline S219 degree 3 poles (-57.0537, 25.5868) (-56.9995, 25.6229) (-56.9529, 25.6693) (-56.8801, 25.7772) (-56.8546, 25.8378) (-56.8326, 25.9437) (-56.8294, 25.9869) (-56.8341, 26.073) (-56.8419, 26.1155) (-56.8552, 26.1565) knots 0 0 0 0 0.019532 0.019532 0.039064 0.039064 0.051994 0.051994 0.064924 0.064924 0.064924 0.064924
  arc A110 (-57.0537, 25.5868) -> (-57.1241, 25.5397) centre (-40, 0) ccw
  spline S220 degree 3 poles (-57.7265, 25.5741) (-57.6769, 25.5319) (-57.6195, 25.4998) (-57.4957, 25.4595) (-57.4304, 25.4516) (-57.3225, 25.4596) (-57.2801, 25.4683) (-57.1987, 25.4965) (-57.1599, 25.5157) (-57.1241, 25.5397) knots 0 0 0 0 0.019532 0.019532 0.039064 0.039064 0.051994 0.051994 0.064924 0.064924 0.064924 0.064924
  spline S221 degree 5 poles (-57.7265, 25.5741) (-57.7278, 25.5753) (-57.7359, 25.5821) (-57.7505, 25.5945) (-57.7719, 25.6125) (-57.8, 25.636) (-57.8337, 25.6638) (-57.8674, 25.6914) (-57.9014, 25.7188) (-57.9355, 25.7461) (-57.9698, 25.7733) (-58.0043, 25.8004) (-58.0389, 25.8273) (-58.0737, 25.854) (-58.1086, 25.8807) (-58.1437, 25.9072) (-58.1789, 25.9335) (-58.2143, 25.9598) (-58.2498, 25.9859) (-58.2855, 26.0118) (-58.3213, 26.0377) (-58.3573, 26.0634) (-58.3934, 26.089) (-58.4296, 26.1144) (-58.466, 26.1398) (-58.5025, 26.165) (-58.5392, 26.1901) (-58.576, 26.215) (-58.6129, 26.2399) (-58.6499, 26.2646) (-58.6871, 26.2892) (-58.7244, 26.3137) (-58.7618, 26.338) (-58.7994, 26.3623) (-58.837, 26.3864) (-58.8748, 26.4104) (-58.9128, 26.4343) (-58.9508, 26.4581) (-58.989, 26.4817) (-59.0273, 26.5053) (-59.0657, 26.5287) (-59.1042, 26.552) (-59.1428, 26.5752) (-59.1815, 26.5983) (-59.2204, 26.6213) (-59.2594, 26.6441) (-59.2985, 26.6669) (-59.3298, 26.685) (-59.3534, 26.6985) (-59.3691, 26.7075) (-59.377, 26.712) knots 0.354152 0.354152 0.354152 0.354152 0.354152 0.354152 0.357143 0.371429 0.385714 0.4 0.414286 0.428571 0.442857 0.457143 0.471429 0.485714 0.5 0.514286 0.528571 0.542857 0.557143 0.571429 0.585714 0.6 0.614286 0.628571 0.642857 0.657143 0.671429 0.685714 0.7 0.714286 0.728571 0.742857 0.757143 0.771429 0.785714 0.8 0.814286 0.828571 0.842857 0.857143 0.871429 0.885714 0.9 0.914286 0.928571 0.942857 0.957143 0.971429 0.985714 1 1 1 1 1 1
  arc A111 (-59.377, 26.712) -> (-59.9484, 26.288) centre (-40, 0) ccw
  spline S222 degree 5 poles (-59.9484, 26.288) (-59.9464, 26.2792) (-59.9424, 26.2615) (-59.9363, 26.235) (-59.928, 26.1998) (-59.9176, 26.1558) (-59.907, 26.1118) (-59.8963, 26.068) (-59.8854, 26.0242) (-59.8744, 25.9805) (-59.8633, 25.9369) (-59.852, 25.8934) (-59.8405, 25.8499) (-59.8289, 25.8065) (-59.8172, 25.7632) (-59.8053, 25.72) (-59.7933, 25.6769) (-59.7812, 25.6338) (-59.7688, 25.5908) (-59.7564, 25.548) (-59.7438, 25.5052) (-59.731, 25.4625) (-59.7181, 25.4198) (-59.705, 25.3773) (-59.6917, 25.3349) (-59.6784, 25.2925) (-59.6648, 25.2503) (-59.6511, 25.2081) (-59.6372, 25.166) (-59.6232, 25.1241) (-59.609, 25.0822) (-59.5947, 25.0404) (-59.5802, 24.9987) (-59.5655, 24.9572) (-59.5506, 24.9157) (-59.5356, 24.8743) (-59.5204, 24.8331) (-59.5051, 24.7919) (-59.4895, 24.7509) (-59.4738, 24.71) (-59.4579, 24.6692) (-59.4419, 24.6285) (-59.4256, 24.5879) (-59.4092, 24.5474) (-59.3925, 24.5071) (-59.3757, 24.4669) (-59.3614, 24.4331) (-59.3504, 24.4074) (-59.3427, 24.3898) (-59.3385, 24.3802) (-59.3378, 24.3785) knots -1 -1 -1 -1 -1 -1 -0.985714 -0.971429 -0.957143 -0.942857 -0.928571 -0.914286 -0.9 -0.885714 -0.871429 -0.857143 -0.842857 -0.828571 -0.814286 -0.8 -0.785714 -0.771429 -0.757143 -0.742857 -0.728571 -0.714286 -0.7 -0.685714 -0.671429 -0.657143 -0.642857 -0.628571 -0.614286 -0.6 -0.585714 -0.571429 -0.557143 -0.542857 -0.528571 -0.514286 -0.5 -0.485714 -0.471429 -0.457143 -0.442857 -0.428571 -0.414286 -0.4 -0.385714 -0.371429 -0.357143 -0.354152 -0.354152 -0.354152 -0.354152 -0.354152 -0.354152
  spline S223 degree 3 poles (-59.4795, 23.7921) (-59.4291, 23.8333) (-59.3873, 23.884) (-59.3254, 23.9986) (-59.3059, 24.0613) (-59.2945, 24.1689) (-59.2955, 24.2122) (-59.3086, 24.2974) (-59.3206, 24.339) (-59.3378, 24.3785) knots 0 0 0 0 0.019532 0.019532 0.039064 0.039064 0.051994 0.051994 0.064924 0.064924 0.064924 0.064924
  arc A112 (-59.4795, 23.7921) -> (-59.545, 23.7383) centre (-40, 0) ccw
  spline S224 degree 3 poles (-60.1478, 23.7135) (-60.0943, 23.6764) (-60.0341, 23.65) (-59.9069, 23.622) (-59.8412, 23.6205) (-59.7346, 23.6391) (-59.6933, 23.6519) (-59.6149, 23.6879) (-59.5783, 23.7109) (-59.545, 23.7383) knots 0 0 0 0 0.019532 0.019532 0.039064 0.039064 0.051994 0.051994 0.064924 0.064924 0.064924 0.064924
  spline S225 degree 5 poles (-60.1478, 23.7135) (-60.1493, 23.7145) (-60.1579, 23.7205) (-60.1737, 23.7314) (-60.1968, 23.7472) (-60.2271, 23.7678) (-60.2633, 23.7922) (-60.2996, 23.8163) (-60.3361, 23.8403) (-60.3727, 23.8642) (-60.4095, 23.8879) (-60.4465, 23.9114) (-60.4835, 23.9348) (-60.5208, 23.958) (-60.5581, 23.9811) (-60.5957, 24.004) (-60.6333, 24.0268) (-60.6711, 24.0494) (-60.709, 24.0719) (-60.7471, 24.0943) (-60.7852, 24.1165) (-60.8235, 24.1385) (-60.862, 24.1605) (-60.9005, 24.1823) (-60.9392, 24.2039) (-60.978, 24.2254) (-61.017, 24.2468) (-61.056, 24.268) (-61.0952, 24.2891) (-61.1345, 24.3101) (-61.1739, 24.331) (-61.2134, 24.3517) (-61.2531, 24.3722) (-61.2928, 24.3927) (-61.3327, 24.413) (-61.3726, 24.4332) (-61.4127, 24.4533) (-61.4529, 24.4732) (-61.4932, 24.493) (-61.5336, 24.5127) (-61.5741, 24.5322) (-61.6147, 24.5516) (-61.6555, 24.5709) (-61.6963, 24.5901) (-61.7372, 24.6092) (-61.7782, 24.6281) (-61.8193, 24.6469) (-61.8523, 24.6619) (-61.8771, 24.673) (-61.8936, 24.6804) (-61.9019, 24.6841) knots 0.354152 0.354152 0.354152 0.354152 0.354152 0.354152 0.357143 0.371429 0.385714 0.4 0.414286 0.428571 0.442857 0.457143 0.471429 0.485714 0.5 0.514286 0.528571 0.542857 0.557143 0.571429 0.585714 0.6 0.614286 0.628571 0.642857 0.657143 0.671429 0.685714 0.7 0.714286 0.728571 0.742857 0.757143 0.771429 0.785714 0.8 0.814286 0.828571 0.842857 0.857143 0.871429 0.885714 0.9 0.914286 0.928571 0.942857 0.957143 0.971429 0.985714 1 1 1 1 1 1
  arc A113 (-61.9019, 24.6841) -> (-62.4291, 24.2061) centre (-40, 0) ccw
  spline S226 degree 5 poles (-62.4291, 24.2061) (-62.4262, 24.1975) (-62.4204, 24.1804) (-62.4117, 24.1546) (-62.4001, 24.1203) (-62.3854, 24.0776) (-62.3705, 24.0349) (-62.3556, 23.9923) (-62.3405, 23.9498) (-62.3252, 23.9074) (-62.3099, 23.8651) (-62.2944, 23.8229) (-62.2787, 23.7807) (-62.2629, 23.7387) (-62.247, 23.6967) (-62.231, 23.6549) (-62.2148, 23.6131) (-62.1985, 23.5715) (-62.182, 23.5299) (-62.1654, 23.4885) (-62.1486, 23.4471) (-62.1317, 23.4059) (-62.1147, 23.3647) (-62.0975, 23.3237) (-62.0802, 23.2827) (-62.0627, 23.2419) (-62.0451, 23.2012) (-62.0273, 23.1606) (-62.0094, 23.1201) (-61.9913, 23.0797) (-61.9731, 23.0394) (-61.9547, 22.9992) (-61.9362, 22.9592) (-61.9175, 22.9192) (-61.8987, 22.8794) (-61.8797, 22.8397) (-61.8605, 22.8002) (-61.8412, 22.7607) (-61.8217, 22.7214) (-61.8021, 22.6822) (-61.7822, 22.6432) (-61.7623, 22.6042) (-61.7421, 22.5654) (-61.7218, 22.5268) (-61.7013, 22.4883) (-61.6806, 22.4499) (-61.663, 22.4177) (-61.6495, 22.3932) (-61.6402, 22.3764) (-61.6351, 22.3673) (-61.6342, 22.3657) knots -1 -1 -1 -1 -1 -1 -0.985714 -0.971429 -0.957143 -0.942857 -0.928571 -0.914286 -0.9 -0.885714 -0.871429 -0.857143 -0.842857 -0.828571 -0.814286 -0.8 -0.785714 -0.771429 -0.757143 -0.742857 -0.728571 -0.714286 -0.7 -0.685714 -0.671429 -0.657143 -0.642857 -0.628571 -0.614286 -0.6 -0.585714 -0.571429 -0.557143 -0.542857 -0.528571 -0.514286 -0.5 -0.485714 -0.471429 -0.457143 -0.442857 -0.428571 -0.414286 -0.4 -0.385714 -0.371429 -0.357143 -0.354152 -0.354152 -0.354152 -0.354152 -0.354152 -0.354152
  spline S227 degree 3 poles (-61.7177, 21.7682) (-61.6717, 21.8141) (-61.635, 21.8687) (-61.5846, 21.9888) (-61.5714, 22.0532) (-61.5706, 22.1614) (-61.5758, 22.2043) (-61.5972, 22.2878) (-61.6132, 22.328) (-61.6342, 22.3657) knots 0 0 0 0 0.019532 0.019532 0.039064 0.039064 0.051994 0.051994 0.064924 0.064924 0.064924 0.064924
  arc A114 (-61.7177, 21.7682) -> (-61.7776, 21.7082) centre (-40, 0) ccw
  spline S228 degree 3 poles (-62.3751, 21.6244) (-62.3182, 21.5928) (-62.2557, 21.5725) (-62.1264, 21.557) (-62.0609, 21.562) (-61.9566, 21.5909) (-61.9167, 21.6078) (-61.8423, 21.6513) (-61.8081, 21.6777) (-61.7776, 21.7082) knots 0 0 0 0 0.019532 0.019532 0.039064 0.039064 0.051994 0.051994 0.064924 0.064924 0.064924 0.064924
  spline S229 degree 5 poles (-62.3751, 21.6244) (-62.3767, 21.6253) (-62.3859, 21.6305) (-62.4027, 21.6398) (-62.4272, 21.6532) (-62.4593, 21.6708) (-62.4977, 21.6915) (-62.5363, 21.7119) (-62.5749, 21.7322) (-62.6137, 21.7524) (-62.6527, 21.7724) (-62.6917, 21.7922) (-62.7309, 21.8118) (-62.7703, 21.8313) (-62.8097, 21.8506) (-62.8493, 21.8697) (-62.889, 21.8887) (-62.9288, 21.9075) (-62.9687, 21.9262) (-63.0088, 21.9447) (-63.049, 21.963) (-63.0893, 21.9812) (-63.1297, 21.9993) (-63.1702, 22.0172) (-63.2108, 22.035) (-63.2515, 22.0526) (-63.2924, 22.07) (-63.3333, 22.0873) (-63.3744, 22.1045) (-63.4155, 22.1215) (-63.4568, 22.1384) (-63.4982, 22.1551) (-63.5396, 22.1717) (-63.5812, 22.1882) (-63.6228, 22.2045) (-63.6646, 22.2207) (-63.7064, 22.2367) (-63.7484, 22.2526) (-63.7904, 22.2683) (-63.8326, 22.284) (-63.8748, 22.2995) (-63.9171, 22.3148) (-63.9595, 22.33) (-64.0021, 22.3451) (-64.0446, 22.3601) (-64.0873, 22.3749) (-64.1301, 22.3896) (-64.1644, 22.4012) (-64.1901, 22.4099) (-64.2073, 22.4156) (-64.2159, 22.4185) knots 0.354152 0.354152 0.354152 0.354152 0.354152 0.354152 0.357143 0.371429 0.385714 0.4 0.414286 0.428571 0.442857 0.457143 0.471429 0.485714 0.5 0.514286 0.528571 0.542857 0.557143 0.571429 0.585714 0.6 0.614286 0.628571 0.642857 0.657143 0.671429 0.685714 0.7 0.714286 0.728571 0.742857 0.757143 0.771429 0.785714 0.8 0.814286 0.828571 0.842857 0.857143 0.871429 0.885714 0.9 0.914286 0.928571 0.942857 0.957143 0.971429 0.985714 1 1 1 1 1 1
  arc A115 (-64.2159, 22.4185) -> (-64.6937, 21.8912) centre (-40, 0) ccw
  spline S230 degree 5 poles (-64.6937, 21.8912) (-64.69, 21.8829) (-64.6826, 21.8663) (-64.6714, 21.8416) (-64.6564, 21.8086) (-64.6376, 21.7675) (-64.6187, 21.7265) (-64.5996, 21.6855) (-64.5804, 21.6447) (-64.5611, 21.604) (-64.5416, 21.5634) (-64.5221, 21.5229) (-64.5024, 21.4825) (-64.4825, 21.4422) (-64.4626, 21.402) (-64.4425, 21.362) (-64.4223, 21.322) (-64.402, 21.2822) (-64.3815, 21.2424) (-64.3609, 21.2028) (-64.3402, 21.1633) (-64.3193, 21.1239) (-64.2983, 21.0846) (-64.2772, 21.0454) (-64.256, 21.0064) (-64.2346, 20.9675) (-64.213, 20.9287) (-64.1914, 20.89) (-64.1696, 20.8514) (-64.1476, 20.813) (-64.1255, 20.7747) (-64.1033, 20.7365) (-64.081, 20.6985) (-64.0585, 20.6606) (-64.0358, 20.6228) (-64.013, 20.5852) (-63.9901, 20.5477) (-63.967, 20.5103) (-63.9437, 20.4731) (-63.9203, 20.436) (-63.8968, 20.3991) (-63.8731, 20.3623) (-63.8492, 20.3257) (-63.8252, 20.2892) (-63.801, 20.2529) (-63.7767, 20.2167) (-63.756, 20.1864) (-63.7402, 20.1634) (-63.7293, 20.1476) (-63.7233, 20.1389) (-63.7223, 20.1374) knots -1 -1 -1 -1 -1 -1 -0.985714 -0.971429 -0.957143 -0.942857 -0.928571 -0.914286 -0.9 -0.885714 -0.871429 -0.857143 -0.842857 -0.828571 -0.814286 -0.8 -0.785714 -0.771429 -0.757143 -0.742857 -0.728571 -0.714286 -0.7 -0.685714 -0.671429 -0.657143 -0.642857 -0.628571 -0.614286 -0.6 -0.585714 -0.571429 -0.557143 -0.542857 -0.528571 -0.514286 -0.5 -0.485714 -0.471429 -0.457143 -0.442857 -0.428571 -0.414286 -0.4 -0.385714 -0.371429 -0.357143 -0.354152 -0.354152 -0.354152 -0.354152 -0.354152 -0.354152
  spline S231 degree 3 poles (-63.7468, 19.5346) (-63.7055, 19.5849) (-63.6743, 19.6428) (-63.636, 19.7672) (-63.6291, 19.8326) (-63.6389, 19.9404) (-63.6483, 19.9826) (-63.6778, 20.0636) (-63.6977, 20.102) (-63.7223, 20.1374) knots 0 0 0 0 0.019532 0.019532 0.039064 0.039064 0.051994 0.051994 0.064924 0.064924 0.064924 0.064924
  arc A116 (-63.7468, 19.5346) -> (-63.8006, 19.4691) centre (-40, 0) ccw
  spline S232 degree 3 poles (-64.3869, 19.3272) (-64.3272, 19.3012) (-64.263, 19.2872) (-64.1328, 19.2845) (-64.0681, 19.2958) (-63.9672, 19.3348) (-63.9291, 19.3555) (-63.8593, 19.4061) (-63.8278, 19.4358) (-63.8006, 19.4691) knots 0 0 0 0 0.019532 0.019532 0.039064 0.039064 0.051994 0.051994 0.064924 0.064924 0.064924 0.064924
  spline S233 degree 5 poles (-64.3869, 19.3272) (-64.3886, 19.3279) (-64.3982, 19.3321) (-64.4159, 19.3397) (-64.4416, 19.3507) (-64.4753, 19.365) (-64.5155, 19.3818) (-64.5559, 19.3985) (-64.5964, 19.4149) (-64.6369, 19.4311) (-64.6776, 19.4472) (-64.7185, 19.463) (-64.7594, 19.4787) (-64.8004, 19.4943) (-64.8416, 19.5096) (-64.8829, 19.5248) (-64.9242, 19.5398) (-64.9657, 19.5546) (-65.0073, 19.5693) (-65.049, 19.5838) (-65.0907, 19.5981) (-65.1326, 19.6123) (-65.1746, 19.6263) (-65.2167, 19.6401) (-65.2588, 19.6538) (-65.3011, 19.6673) (-65.3435, 19.6807) (-65.3859, 19.6939) (-65.4284, 19.707) (-65.4711, 19.7199) (-65.5138, 19.7326) (-65.5566, 19.7452) (-65.5995, 19.7577) (-65.6424, 19.77) (-65.6855, 19.7821) (-65.7286, 19.7941) (-65.7719, 19.806) (-65.8152, 19.8177) (-65.8586, 19.8292) (-65.902, 19.8407) (-65.9456, 19.8519) (-65.9892, 19.8631) (-66.0329, 19.874) (-66.0767, 19.8849) (-66.1205, 19.8956) (-66.1645, 19.9062) (-66.2085, 19.9166) (-66.2437, 19.9248) (-66.2702, 19.9309) (-66.2879, 19.935) (-66.2967, 19.937) knots 0.354152 0.354152 0.354152 0.354152 0.354152 0.354152 0.357143 0.371429 0.385714 0.4 0.414286 0.428571 0.442857 0.457143 0.471429 0.485714 0.5 0.514286 0.528571 0.542857 0.557143 0.571429 0.585714 0.6 0.614286 0.628571 0.642857 0.657143 0.671429 0.685714 0.7 0.714286 0.728571 0.742857 0.757143 0.771429 0.785714 0.8 0.814286 0.828571 0.842857 0.857143 0.871429 0.885714 0.9 0.914286 0.928571 0.942857 0.957143 0.971429 0.985714 1 1 1 1 1 1
  arc A117 (-66.2967, 19.937) -> (-66.7205, 19.3653) centre (-40, 0) ccw
  spline S234 degree 5 poles (-66.7205, 19.3653) (-66.716, 19.3575) (-66.707, 19.3417) (-66.6934, 19.3182) (-66.6753, 19.2868) (-66.6525, 19.2477) (-66.6297, 19.2088) (-66.6067, 19.1699) (-66.5836, 19.1312) (-66.5604, 19.0926) (-66.537, 19.0541) (-66.5136, 19.0157) (-66.49, 18.9774) (-66.4664, 18.9393) (-66.4426, 18.9012) (-66.4187, 18.8633) (-66.3946, 18.8255) (-66.3705, 18.7879) (-66.3462, 18.7503) (-66.3219, 18.7129) (-66.2974, 18.6756) (-66.2727, 18.6385) (-66.248, 18.6014) (-66.2231, 18.5645) (-66.1982, 18.5277) (-66.173, 18.4911) (-66.1478, 18.4546) (-66.1225, 18.4182) (-66.097, 18.382) (-66.0714, 18.3459) (-66.0457, 18.31) (-66.0198, 18.2741) (-65.9938, 18.2385) (-65.9677, 18.203) (-65.9414, 18.1676) (-65.9151, 18.1324) (-65.8886, 18.0973) (-65.8619, 18.0624) (-65.8351, 18.0276) (-65.8082, 17.993) (-65.7812, 17.9586) (-65.754, 17.9243) (-65.7266, 17.8902) (-65.6992, 17.8562) (-65.6715, 17.8225) (-65.6438, 17.7888) (-65.6203, 17.7607) (-65.6023, 17.7393) (-65.5898, 17.7247) (-65.583, 17.7167) (-65.5818, 17.7153) knots -1 -1 -1 -1 -1 -1 -0.985714 -0.971429 -0.957143 -0.942857 -0.928571 -0.914286 -0.9 -0.885714 -0.871429 -0.857143 -0.842857 -0.828571 -0.814286 -0.8 -0.785714 -0.771429 -0.757143 -0.742857 -0.728571 -0.714286 -0.7 -0.685714 -0.671429 -0.657143 -0.642857 -0.628571 -0.614286 -0.6 -0.585714 -0.571429 -0.557143 -0.542857 -0.528571 -0.514286 -0.5 -0.485714 -0.471429 -0.457143 -0.442857 -0.428571 -0.414286 -0.4 -0.385714 -0.371429 -0.357143 -0.354152 -0.354152 -0.354152 -0.354152 -0.354152 -0.354152
  spline S235 degree 3 poles (-65.5472, 17.113) (-65.511, 17.1671) (-65.4856, 17.2277) (-65.4597, 17.3553) (-65.4593, 17.421) (-65.4796, 17.5273) (-65.4931, 17.5684) (-65.5303, 17.6462) (-65.5539, 17.6825) (-65.5818, 17.7153) knots 0 0 0 0 0.019532 0.019532 0.039064 0.039064 0.051994 0.051994 0.064924 0.064924 0.064924 0.064924
  arc A118 (-65.5472, 17.113) -> (-65.5943, 17.0425) centre (-40, 0) ccw
  spline S236 degree 3 poles (-66.1639, 16.8438) (-66.1019, 16.8238) (-66.0367, 16.8161) (-65.9068, 16.8262) (-65.8435, 16.8438) (-65.7469, 16.8925) (-65.7111, 16.9168) (-65.6466, 16.974) (-65.6181, 17.0066) (-65.5943, 17.0425) knots 0 0 0 0 0.019532 0.019532 0.039064 0.039064 0.051994 0.051994 0.064924 0.064924 0.064924 0.064924
  spline S237 degree 5 poles (-66.1639, 16.8438) (-66.1656, 16.8443) (-66.1756, 16.8476) (-66.1939, 16.8534) (-66.2206, 16.8619) (-66.2556, 16.8728) (-66.2972, 16.8856) (-66.339, 16.8981) (-66.3809, 16.9105) (-66.4229, 16.9227) (-66.465, 16.9347) (-66.5072, 16.9465) (-66.5494, 16.9581) (-66.5918, 16.9695) (-66.6343, 16.9808) (-66.6768, 16.9918) (-66.7194, 17.0027) (-66.7622, 17.0134) (-66.805, 17.0239) (-66.8479, 17.0342) (-66.8909, 17.0444) (-66.9339, 17.0544) (-66.9771, 17.0642) (-67.0203, 17.0739) (-67.0636, 17.0834) (-67.107, 17.0927) (-67.1505, 17.1018) (-67.194, 17.1108) (-67.2376, 17.1196) (-67.2813, 17.1283) (-67.3251, 17.1368) (-67.3689, 17.1452) (-67.4128, 17.1533) (-67.4568, 17.1614) (-67.5008, 17.1692) (-67.5449, 17.177) (-67.5891, 17.1845) (-67.6333, 17.1919) (-67.6777, 17.1992) (-67.722, 17.2063) (-67.7665, 17.2132) (-67.811, 17.22) (-67.8555, 17.2267) (-67.9002, 17.2332) (-67.9449, 17.2395) (-67.9896, 17.2457) (-68.0344, 17.2518) (-68.0703, 17.2565) (-68.0973, 17.26) (-68.1153, 17.2623) (-68.1243, 17.2634) knots 0.354152 0.354152 0.354152 0.354152 0.354152 0.354152 0.357143 0.371429 0.385714 0.4 0.414286 0.428571 0.442857 0.457143 0.471429 0.485714 0.5 0.514286 0.528571 0.542857 0.557143 0.571429 0.585714 0.6 0.614286 0.628571 0.642857 0.657143 0.671429 0.685714 0.7 0.714286 0.728571 0.742857 0.757143 0.771429 0.785714 0.8 0.814286 0.828571 0.842857 0.857143 0.871429 0.885714 0.9 0.914286 0.928571 0.942857 0.957143 0.971429 0.985714 1 1 1 1 1 1
  arc A119 (-68.1243, 17.2634) -> (-68.4899, 16.653) centre (-40, 0) ccw
  spline S238 degree 5 poles (-68.4899, 16.653) (-68.4847, 16.6456) (-68.4742, 16.6309) (-68.4584, 16.6087) (-68.4373, 16.5793) (-68.4108, 16.5427) (-68.3842, 16.5061) (-68.3575, 16.4697) (-68.3308, 16.4334) (-68.3039, 16.3973) (-68.2769, 16.3612) (-68.2498, 16.3253) (-68.2226, 16.2896) (-68.1953, 16.2539) (-68.1679, 16.2184) (-68.1404, 16.183) (-68.1128, 16.1478) (-68.085, 16.1126) (-68.0572, 16.0777) (-68.0293, 16.0428) (-68.0013, 16.0081) (-67.9731, 15.9735) (-67.9449, 15.9391) (-67.9165, 15.9048) (-67.888, 15.8707) (-67.8595, 15.8367) (-67.8308, 15.8028) (-67.802, 15.7691) (-67.7731, 15.7355) (-67.7441, 15.7021) (-67.7149, 15.6689) (-67.6857, 15.6358) (-67.6563, 15.6028) (-67.6269, 15.57) (-67.5973, 15.5374) (-67.5676, 15.5049) (-67.5377, 15.4726) (-67.5078, 15.4405) (-67.4777, 15.4085) (-67.4476, 15.3767) (-67.4173, 15.3451) (-67.3868, 15.3137) (-67.3563, 15.2824) (-67.3256, 15.2513) (-67.2948, 15.2204) (-67.2639, 15.1897) (-67.2377, 15.164) (-67.2177, 15.1445) (-67.2039, 15.1311) (-67.1964, 15.1238) (-67.1951, 15.1225) knots -1 -1 -1 -1 -1 -1 -0.985714 -0.971429 -0.957143 -0.942857 -0.928571 -0.914286 -0.9 -0.885714 -0.871429 -0.857143 -0.842857 -0.828571 -0.814286 -0.8 -0.785714 -0.771429 -0.757143 -0.742857 -0.728571 -0.714286 -0.7 -0.685714 -0.671429 -0.657143 -0.642857 -0.628571 -0.614286 -0.6 -0.585714 -0.571429 -0.557143 -0.542857 -0.528571 -0.514286 -0.5 -0.485714 -0.471429 -0.457143 -0.442857 -0.428571 -0.414286 -0.4 -0.385714 -0.371429 -0.357143 -0.354152 -0.354152 -0.354152 -0.354152 -0.354152 -0.354152
  spline S239 degree 3 poles (-67.1015, 14.5265) (-67.0708, 14.5839) (-67.0515, 14.6467) (-67.0382, 14.7763) (-67.0442, 14.8417) (-67.0749, 14.9455) (-67.0923, 14.9851) (-67.137, 15.0588) (-67.164, 15.0926) (-67.1951, 15.1225) knots 0 0 0 0 0.019532 0.019532 0.039064 0.039064 0.051994 0.051994 0.064924 0.064924 0.064924 0.064924
  arc A120 (-67.1015, 14.5265) -> (-67.1415, 14.4518) centre (-40, 0) ccw
  spline S240 degree 3 poles (-67.6889, 14.1982) (-67.6253, 14.1843) (-67.5595, 14.1831) (-67.4313, 14.2058) (-67.3701, 14.2296) (-67.2787, 14.2876) (-67.2454, 14.3153) (-67.1868, 14.3785) (-67.1617, 14.4137) (-67.1415, 14.4518) knots 0 0 0 0 0.019532 0.019532 0.039064 0.039064 0.051994 0.051994 0.064924 0.064924 0.064924 0.064924